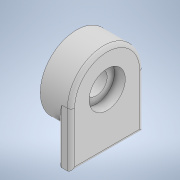
# Autodesk Inventor part: base8
Saved by Autodesk Inventor 2022 (Build 260153000, 153)
## iProperties
Created: 2022-06-14
Part Number: base8
Material: 一般
Document SubType Name: Modeling
Designer: yuto6
Density: 1 g/cm^3
Appearance: 既定
Author: yuto6
Autodesk Inventor part; units mm, degrees
ref_plane "YZ Plane" through (0, 0, 0) normal (1, 0, 0) x (0, 1, 0)
ref_plane "XZ Plane" through (0, 0, 0) normal (0, 1, 0) x (-1, 0, 0)
ref_plane "XY Plane" through (0, 0, 0) normal (0, 0, 1) x (1, 0, 0)
sketch "スケッチ1" plane through (0, 0, 0) normal (1, 0, 0) x (0, 1, 0)
  circle A0 centre (0, 0) radius 10
  line L0 (0, 10) -> (-15, 10)
  line L1 (-15, 10) -> (-15, -10)
  line L2 (-15, -10) -> (0, -10)
  line L3 (0, -10) -> (0, 10)
  dimension "d0" = 20
  dimension "d1" = 15
  constraints: 8 end point, 3 horizontal, 2 parallel, 1 coincident, 1 perpendicular, 3 other
  measures "d1" distance of L0.start L0.end
extrude "押し出し1" add sketch "スケッチ1" along normal blind 3.5
hole "穴1" at (0, 0, 0) direction (1, 0, 0) diameter 6 end through all
sketch "スケッチ3" plane through (0, 0, 0) normal (-1, 0, 0) x (0, 0, 1)
  circle A0 centre (0, 0) radius 3 projected
  circle A1 centre (0, 0) radius 10
  constraints: 1 centre point, 1 coincident
extrude "押し出し3" add sketch "スケッチ3" along normal blind 5
sketch "スケッチ4" plane through (3.5, 0, 0) normal (1, 0, 0) x (0, 0, -1)
  circle A0 centre (0, 0) radius 5
  dimension "d19" = 10
  constraints: 1 centre point, 1 coincident
  measures "d19" diameter of A0
extrude "押し出し4" cut sketch "スケッチ4" against normal blind 3
sketch "スケッチ5" plane through (-5, 0, 0) normal (-1, 0, 0) x (0, 0, 1)
  circle A0 centre (0, 0) radius 4
  circle A1 centre (0, 0) radius 3
  dimension "d22" = 8
  constraints: 2 centre point, 2 coincident
  measures "d22" diameter of A0
extrude "押し出し5" add sketch "スケッチ5" along normal blind 1
fillet "フィレット3" radius 1 1 edges at (-5, 0, -4)
fillet "フィレット4" radius 1 7 edges at (3.5, -7.5, 10) (3.5, -7.5, -10) (3.5, 10, 0) (0, -7.5, 10) (3.5, -15, 0) (0, -15, 0) (0, -7.5, -10)
sketch "スケッチ2" plane through (0, 0, 0) normal (-1, 0, 0) x (0, 0, 1)
  circle A0 centre (0, 0) radius 3
  circle A1 centre (0, 0) radius 4
  dimension "d11" = 8
  dimension "d12" = 6
  constraints: 2 centre point, 2 coincident
  measures "d11" diameter of A1
  measures "d12" diameter of A0
